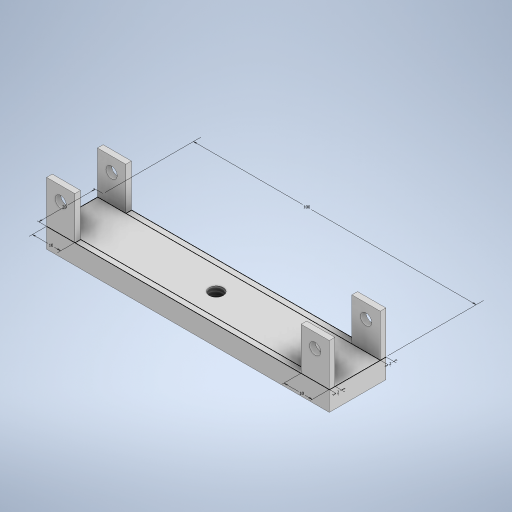
# Autodesk Inventor part: RadarMount
Saved by Autodesk Inventor 2023 (Build 270158000, 158)
## iProperties
Created: 2023-07-19
Part Number: RadarMount
Material: Generic
Document SubType Name: Modeling
Designer: beckb
Density: 1 g/cm^3
Appearance: Default
Author: beckb
Autodesk Inventor part; units mm, degrees
ref_plane "YZ Plane" through (0, 0, 0) normal (1, 0, 0) x (0, 1, 0)
ref_plane "XZ Plane" through (0, 0, 0) normal (0, 1, 0) x (-1, 0, 0)
ref_plane "XY Plane" through (0, 0, 0) normal (0, 0, 1) x (1, 0, 0)
sketch "Sketch1" plane through (0, 0, 0) normal (0, 1, 0) x (-1, 0, 0)
  line L0 (0, 0) -> (100, 0)
  line L1 (100, 0) -> (100, -20)
  line L2 (100, -20) -> (0, -20)
  line L3 (0, -20) -> (0, 0)
  line L4 (100, -2) -> (0, -2)
  line L5 (100, -18) -> (0, -18)
  line L6 (10, 0) -> (10, -2)
  line L7 (10, -18) -> (10, -20)
  line L8 (90, 0) -> (90, -2)
  line L9 (90, -18) -> (90, -20)
  dimension "d0" = 20
  dimension "d1" = 100
  dimension "d2" = 2
  dimension "d3" = 2
  dimension "d5" = 10
  dimension "d6" = 10
  constraints: 20 end point, 16 point on line, 5 perpendicular, 2 parallel, 1 horizontal
  measures "d0" distance of L0.end L1.end
  measures "d1" distance of L1.end L2.end
  measures "d2" distance between parallel lines of L2 L5
  measures "d3" distance between parallel lines of L0 L4
  measures "d5" distance between parallel lines of L3 L6
  measures "d6" distance between parallel lines of L8 L1
extrude "Extrusion1" add sketch "Sketch1" along normal blind 15 contours L0 L6 L4 L3 | L0 L1 L4 L8 | L5 L7 L2 L3 | L5 L1 L2 L9
extrude "Extrusion2" add sketch "Sketch1" against normal blind 7
sketch "Sketch2" plane through (-10, 15, 0) normal (0, 0, 1) x (1, 0, 0)
  circle A0 centre (5, -5) radius 2
  line L0 (10, -22) -> (10, 0) projected
  line L1 (0, 0) -> (10, 0) projected
  circle A1 centre (-85, -5) radius 2
  line L2 (-80, -15) -> (-80, 0) projected
  line L3 (-90, 0) -> (-80, 0) projected
  point P0 (10, -15)
  dimension "d11" = 4
  dimension "d12" = 5
  dimension "d13" = 5
  dimension "d14" = 4
  dimension "d15" = 5
  dimension "d16" = 5
  constraints: 2 centre point
  measures "d11" diameter of A0
  measures "d12" distance from line of L0 A0.centre
  measures "d13" distance from line of L1 A0.centre
  measures "d14" diameter of A1
  measures "d15" distance from line of L2 A1.centre
  measures "d16" distance from line of L3 A1.centre
sketch "Sketch3" plane through (0, 15, -20) normal (0, 0, -1) x (-1, 0, 0)
  circle A0 centre (5, -5) radius 2
  line L0 (10, -15) -> (10, 0) projected
  line L1 (0, 0) -> (10, 0) projected
  circle A1 centre (95, -5) radius 2
  line L2 (90, 0) -> (100, 0) projected
  line L3 (100, -22) -> (100, 0) projected
  point P0 (0, -15)
  dimension "d17" = 4
  dimension "d18" = 5
  dimension "d19" = 5
  dimension "d20" = 4
  dimension "d21" = 5
  dimension "d22" = 5
  constraints: 2 centre point
  measures "d17" diameter of A0
  measures "d18" distance from line of L0 A0.centre
  measures "d19" distance from line of L1 A0.centre
  measures "d20" diameter of A1
  measures "d21" distance from line of A1.centre L2
  measures "d22" distance from line of L3 A1.centre
extrude "Extrusion3" cut sketch "Sketch3" against normal blind 7
extrude "Extrusion4" cut sketch "Sketch2" against normal blind 7
sketch "Sketch4" plane through (0, -7, 0) normal (0, -1, 0) x (1, 0, 0)
  line L0 (-100, -20) -> (0, -20) projected
  line L1 (-100, 0) -> (-100, -20) projected
  point P0 (0, 0)
  point P1 (-50, -10)
  dimension "d27" = 10
  dimension "d28" = 50
  measures "d27" distance from line of L0 point (-50, -10)
  measures "d28" distance from line of L1 point (-50, -10)
hole "Hole1" at (-50, -7, -10) direction (0, 1, 0) diameter 4.9784 end through all thread size "1/4-20 UNC" class "1B" standard "ANSI Unified Screw Threads"
body "Solid1"
